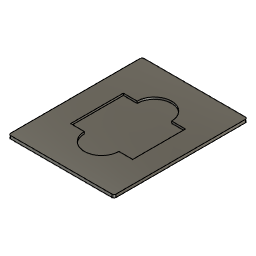
Wingspan - Bonus Cards Lid (Autodesk Fusion 360 design; units mm, degrees)
Autodesk Fusion 360 part; units mm, degrees
sketch "Skizze1" plane through (0, 0, 0) normal (0, 0, 1) x (1, 0, 0)
  line L0 (0, 0) -> (107, 0)
  line L1 (107, 0) -> (107, 135.5)
  line L2 (107, 135.5) -> (0, 135.5)
  line L3 (0, 135.5) -> (0, 0)
  dimension "d1" = 107
  dimension "d2" = 135.5
  constraint horizontal L0
  constraint vertical L1
  constraint horizontal L2
  constraint vertical L3
  constraint coincident L0.start L3.end
  measures "d1" distance of L0.start L0.end
  measures "d2" distance of L0.start L2.end
extrude "Extrusion1" add sketch "Skizze1" along normal blind 3
sketch "Skizze2" plane through (0, 0, 3) normal (0, 0, 1) x (-1, 0, 0)
  line L0 (0, -135.5) -> (0, 0)
  line L1 (0, 0) -> (-107, 0)
  line L2 (-107, 0) -> (-107, -135.5)
  line L3 (-107, -135.5) -> (0, -135.5)
  line L4 (-22, -41) -> (-85, -41)
  line L5 (-85, -41) -> (-85, -94.5)
  line L6 (-85, -94.5) -> (-22, -94.5)
  line L7 (-22, -94.5) -> (-22, -41)
  circle A0 centre (-53.5, -41) radius 17.5
  circle A1 centre (-53.5, -94.5) radius 17.5
  dimension "d5" = 63
  dimension "d6" = 53.5
  dimension "d7" = 41
  dimension "d8" = 22
  dimension "d9" = 35
  dimension "d10" = 35
  constraint horizontal L4
  constraint vertical L5
  constraint horizontal L6
  constraint vertical L7
  constraint midpoint L4 A0.centre
  constraint midpoint L6 A1.centre
  measures "d5" distance of L4.start L4.end
  measures "d6" distance of L4.start L6.end
  measures "d7" distance of L1 L4
  measures "d8" distance of L2 L5
  measures "d9" diameter of A0
  measures "d10" diameter of A1
extrude "Extrusion2" cut sketch "Skizze2" against normal blind 2 contours L4 L5 L6 L7 A0 A1 | L4 A0 | L4 A0 | L6 A1 | L6 A1
sketch "Skizze3" plane through (0, 0, 0) normal (0, 0, -1) x (1, 0, 0)
  line L0 (0, 0) -> (0, -135.5)
  line L1 (0, -135.5) -> (107, -135.5)
  line L2 (107, -135.5) -> (107, 0)
  line L3 (107, 0) -> (0, 0)
  line L4 (0, 0) -> (7, 0)
  line L5 (7, 0) -> (7, -7)
  line L6 (7, -7) -> (0, -7)
  line L7 (0, -7) -> (0, 0)
  line L8 (107, 0) -> (100, 0)
  line L9 (100, 0) -> (100, -7)
  line L10 (100, -7) -> (107, -7)
  line L11 (107, -7) -> (107, 0)
  line L12 (0, -135.5) -> (7, -135.5)
  line L13 (7, -135.5) -> (7, -128.5)
  line L14 (7, -128.5) -> (0, -128.5)
  line L15 (0, -128.5) -> (0, -135.5)
  line L16 (107, -135.5) -> (100, -135.5)
  line L17 (100, -135.5) -> (100, -128.5)
  line L18 (100, -128.5) -> (107, -128.5)
  line L19 (107, -128.5) -> (107, -135.5)
  circle A0 centre (3.5, -132) radius 2.65
  circle A1 centre (103.5, -132) radius 2.65
  circle A2 centre (103.5, -3.5) radius 2.65
  circle A3 centre (3.5, -3.5) radius 2.65
  dimension "d13" = 7
  dimension "d14" = 7
  dimension "d15" = 7
  dimension "d16" = 7
  dimension "d17" = 7
  dimension "d18" = 7
  dimension "d19" = 7
  dimension "d20" = 7
  dimension "d21" = 5.3
  dimension "d22" = 5.3
  dimension "d23" = 5.3
  dimension "d24" = 5.3
  dimension "d25" = 3.5
  dimension "d26" = 3.5
  dimension "d27" = 3.5
  dimension "d28" = 3.5
  dimension "d29" = 3.5
  dimension "d30" = 3.5
  dimension "d31" = 3.5
  dimension "d32" = 3.5
  constraint horizontal L4
  constraint vertical L5
  constraint horizontal L6
  constraint vertical L7
  constraint coincident L0.start L3.end
  constraint horizontal L8
  constraint vertical L9
  constraint horizontal L10
  constraint vertical L11
  constraint coincident L2.end L3.start
  constraint horizontal L12
  constraint vertical L13
  constraint horizontal L14
  constraint vertical L15
  constraint coincident L0.end L1.start
  constraint horizontal L16
  constraint vertical L17
  constraint horizontal L18
  constraint vertical L19
  constraint coincident L1.end L2.start
  measures "d13" distance of L0.start L4.end
  measures "d14" distance of L0.start L6.end
  measures "d15" distance of L2.end L8.end
  measures "d16" distance of L2.end L10.end
  measures "d17" distance of L0.end L12.end
  measures "d18" distance of L0.end L14.end
  measures "d19" distance of L1.end L16.end
  measures "d20" distance of L1.end L18.end
  measures "d21" diameter of A0
  measures "d22" diameter of A1
  measures "d23" diameter of A2
  measures "d24" diameter of A3
  measures "d25" distance of L7 A3.centre
  measures "d26" distance of L4 A3.centre
  measures "d27" distance of L8 A2.centre
  measures "d28" distance of L11 A2.centre
  measures "d29" distance of L18 A1.centre
  measures "d30" distance of L19 A1.centre
  measures "d31" distance of L13 A0.centre
  measures "d32" distance of L14 A0.centre
extrude "Extrusion3" cut sketch "Skizze3" against normal blind 1.2 contours A0 | A1 | A2 | A3
fillet "Abrundung1" radius 2 4 edges at (107, 0, 1.5) (107, 135.5, 1.5) (0, 135.5, 1.5) (0, 0, 1.5)
equation "d7 = 44 mm - 3 mm"
